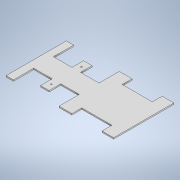
# Autodesk Inventor part: onderkant
Saved by Autodesk Inventor 2022 (Build 260153000, 153)
## iProperties
Created: 2021-12-16
Part Number: onderkant
Material: Generic
Document SubType Name: Modeling
Designer: keemi
Density: 1 g/cm^3
Appearance: Default
Author: keemi
Autodesk Inventor part; units mm, degrees
ref_plane "YZ Plane" through (0, 0, 0) normal (1, 0, 0) x (0, 1, 0)
ref_plane "XZ Plane" through (0, 0, 0) normal (0, 1, 0) x (-1, 0, 0)
ref_plane "XY Plane" through (0, 0, 0) normal (0, 0, 1) x (1, 0, 0)
sketch "Sketch1" plane through (0, 0, 0) normal (0, 1, 0) x (-1, 0, 0)
  line L0 (0, 0) -> (250, 0)
  line L1 (250, 0) -> (250, -140)
  line L2 (250, -140) -> (0, -140)
  line L3 (0, -140) -> (0, 0)
  dimension "d0" = 250
  dimension "d1" = 140
  constraints: 8 end point, 2 parallel, 1 horizontal, 1 perpendicular
  measures "d0" distance of L1.end L2.end
  measures "d1" distance of L0.end L1.end
extrude "Extrusion1" add sketch "Sketch1" along normal blind 3
sketch "Sketch2" plane through (0, 3, 0) normal (0, 1, 0) x (1, 0, 0)
  line L0 (-250, 140) -> (-250, 0) projected
  line L1 (-250, 0) -> (-180, 0)
  line L2 (-250, 0) -> (0, 0) projected
  line L3 (-180, 0) -> (-180, 20)
  line L4 (-180, 0) -> (-170, 0)
  line L5 (-170, 0) -> (-190, 0)
  line L6 (-190, 0) -> (-190, 20)
  line L7 (-190, 20) -> (-170, 20)
  line L8 (-170, 20) -> (-170, 0)
  line L9 (-190, 0) -> (-233, 0)
  line L10 (-233, 0) -> (-233, 47)
  line L11 (-233, 47) -> (-190, 47)
  line L12 (-190, 47) -> (-190, 0)
  line L13 (-170, 0) -> (-127, 0)
  line L14 (-127, 0) -> (-127, 47)
  line L15 (-127, 47) -> (-170, 47)
  line L16 (-170, 47) -> (-170, 0)
  line L17 (-190, 47) -> (-190, 140)
  line L18 (0, 140) -> (-250, 140) projected
  line L19 (-190, 140) -> (-233, 140)
  line L20 (-233, 140) -> (-233, 93)
  line L21 (-233, 93) -> (-190, 93)
  line L22 (-190, 93) -> (-190, 140)
  line L23 (-190, 140) -> (-170, 140)
  line L24 (-170, 140) -> (-170, 120)
  line L25 (-170, 120) -> (-190, 120)
  line L26 (-190, 120) -> (-190, 140)
  line L27 (-170, 140) -> (-127, 140)
  line L28 (-127, 140) -> (-127, 93)
  line L29 (-127, 93) -> (-170, 93)
  line L30 (-170, 93) -> (-170, 140)
  point P0 (-190, 20)
  point P1 (-233, 0)
  point P2 (-127, 0)
  point P3 (-127, 140)
  point P4 (-233, 140)
  point P5 (-190, 93)
  point P6 (-170, 140)
  point P7 (-190, 0)
  point P8 (-180, 20)
  dimension "d4" = 70
  dimension "d5" = 20
  dimension "d6" = 10
  dimension "d7" = 20
  dimension "d8" = 20
  dimension "d9" = 43
  dimension "d10" = 47
  dimension "d11" = 43
  dimension "d12" = 47
  dimension "d31" = 43
  dimension "d32" = 47
  dimension "d33" = 20
  dimension "d34" = 20
  dimension "d35" = 43
  dimension "d36" = 47
  constraints: 56 end point, 12 parallel, 7 perpendicular, 6 horizontal, 3 point on line, 1 vertical
  measures "d4" distance of L0.end L1.end
  measures "d5" distance of L1.end L3.end
  measures "d6" distance of L1.end L4.end
  measures "d7" distance of L6.end L7.end
  measures "d8" distance of L5.end L6.end
  measures "d9" distance of L10.end L11.end
  measures "d10" distance of L9.end L10.end
  measures "d11" distance of L15.end L14.end
  measures "d12" distance of L14.end L13.end
  measures "d31" distance of L21.end L20.end
  measures "d32" distance of L20.end L19.end
  measures "d33" distance of L24.end L25.end
  measures "d34" distance of L23.end L24.end
  measures "d35" distance of L28.end L29.end
  measures "d36" distance of L27.end L28.end
extrude "Extrusion2" cut sketch "Sketch2" against normal blind 50 contours L18 L17 L21 L20 | L10 L11 L12 L6 L1 | L18 L24 L25 L17 | L6 L7 L3 L1 | L18 L28 L29 L30 L24 | L3 L7 L8 L2 | L8 L16 L15 L14 L2
sketch "Sketch3" plane through (0, 3, 0) normal (0, 1, 0) x (1, 0, 0)
  line L0 (-190, 20) -> (-190, 47) projected
  line L1 (-190, 20) -> (-180, 20)
  line L2 (-190, 20) -> (-170, 20) projected
  line L3 (-180, 20) -> (-180, 35)
  line L4 (-190, 120) -> (-190, 93) projected
  line L5 (-190, 120) -> (-180, 120)
  line L6 (-170, 120) -> (-190, 120) projected
  line L7 (-180, 120) -> (-180, 105)
  point P0 (0, 0)
  dimension "d21" = 15
  dimension "d43" = 10
  dimension "d44" = 15
  constraints: 8 end point, 2 midpoint, 1 perpendicular, 1 vertical
  measures "d21" distance of L1.end L3.end
  measures "d43" distance of L4.start L5.end
  measures "d44" distance of L5.end L7.end
hole "Hole1" at (-180, 3, -35) at (-180, 3, -105) direction (0, -1, 0) diameter 3 end through all
sketch "Sketch5" plane through (0, 3, 0) normal (0, 1, 0) x (1, 0, 0)
  line L0 (0, 140) -> (-127, 140) projected
  line L1 (0, 140) -> (-27, 140)
  line L2 (-27, 140) -> (-97, 140)
  line L3 (-97, 140) -> (-97, 117)
  line L4 (-97, 117) -> (-27, 117)
  line L5 (-27, 117) -> (-27, 140)
  line L6 (-27, 140) -> (-27, 0)
  line L7 (-127, 0) -> (0, 0) projected
  line L8 (-27, 0) -> (-97, 0)
  line L9 (-97, 0) -> (-97, 23)
  line L10 (-97, 23) -> (-27, 23)
  line L11 (-27, 23) -> (-27, 0)
  dimension "d45" = 27
  dimension "d46" = 70
  dimension "d47" = 23
  dimension "d48" = 70
  dimension "d49" = 23
  constraints: 20 end point, 4 parallel, 2 horizontal, 2 perpendicular, 2 point on line, 1 vertical
  measures "d45" distance of L0.start L1.end
  measures "d46" distance of L4.end L3.end
  measures "d47" distance of L3.end L2.end
  measures "d48" distance of L9.end L10.end
  measures "d49" distance of L8.end L9.end
extrude "Extrusion4" cut sketch "Sketch5" against normal blind 50
equation "\"d9\" = d11"
equation "\"d10\" = d12"
equation "\"d31\" = d35"
equation "\"d32\" = d36"
equation "\"d35\" = d11"
equation "\"d36\" = d12"
equation "\"d13\" = d16"
equation "\"d50\" = d16"
equation "\"d16\" = 50"
body "Solid1"
